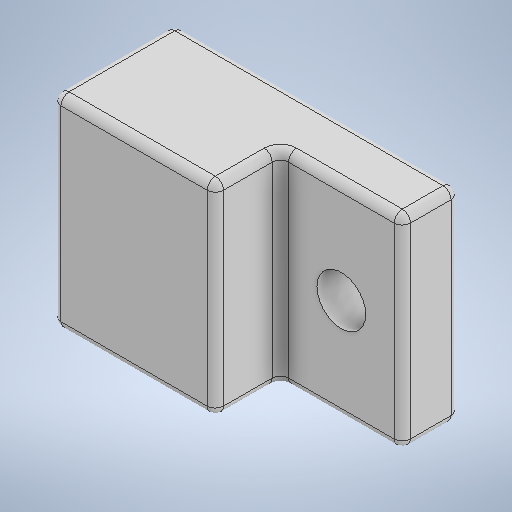
# Autodesk Inventor part: Holder
Saved by Autodesk Inventor 2025.1 (Build 291241000, 241)
## iProperties
Created: 2024-11-13
Part Number: Holder
Material: Genérico
Document SubType Name: Modeling
Designer: feror
Density: 1 g/cm^3
Appearance: Valor por defecto
Author: feror
Autodesk Inventor part; units mm, degrees
ref_plane "YZ Plane" through (0, 0, 0) normal (1, 0, 0) x (0, 1, 0)
ref_plane "XZ Plane" through (0, 0, 0) normal (0, 1, 0) x (-1, 0, 0)
ref_plane "XY Plane" through (0, 0, 0) normal (0, 0, 1) x (1, 0, 0)
sketch "Boceto1" plane through (0, 0, 0) normal (0, 0, 1) x (1, 0, 0)
  line L0 (0, 0) -> (35, 0)
  line L1 (35, 0) -> (35, 25)
  line L2 (35, 25) -> (0, 25)
  line L3 (0, 25) -> (0, 0)
  dimension "d0" = 35
  dimension "d1" = 25
  constraints: 8 end point, 2 parallel, 1 horizontal, 1 perpendicular
  measures "d0" distance of L2.end L1.end
  measures "d1" distance of L1.end L0.end
extrude "Extrusión1" add sketch "Boceto1" along normal blind 15
sketch "Boceto2" plane through (0, 0, 15) normal (0, 0, 1) x (1, 0, 0)
  line L0 (35, 0) -> (35, 25) projected
  line L1 (35, 25) -> (0, 25) projected
  line L2 (35, 0) -> (20, 0)
  line L3 (20, 0) -> (20, 25)
  line L4 (20, 25) -> (35, 25)
  line L5 (35, 25) -> (35, 0)
  point P0 (0, 0)
  dimension "d4" = 15
  constraints: 8 end point, 2 parallel, 1 horizontal, 1 perpendicular, 1 point on line
  measures "d4" distance of L3.end L4.end
extrude "Extrusión2" cut sketch "Boceto2" against normal blind 8
fillet "Empalme1" radius 1 18 edges at (20, 25, 11) (20, 12.5, 15) (27.5, 25, 7) (20, 12.5, 7) (35, 12.5, 7) (35, 25, 3.5) (35, 12.5, 0) (17.5, 25, 0) (10, 25, 15) (0, 25, 7.5) (0, 12.5, 15) (10, 0, 15) (20, 0, 11) (27.5, 0, 7) (35, 0, 3.5) (17.5, 0, 0) (0, 0, 7.5) (0, 12.5, 0)
sketch "Boceto3" plane through (0, 0, 7) normal (0, 0, 1) x (1, 0, 0)
  point P0 (0, 0)
sketch "Boceto4" plane through (0, 0, 7) normal (0, 0, 1) x (1, 0, 0)
  line L0 (21, 24) -> (34, 24) projected
  line L1 (27.5, 24) -> (27.5, 12.5)
  line L2 (27.5, 12.5) -> (34, 12.5)
  circle A0 centre (27.5, 12.5) radius 3
  point P0 (0, 0)
  dimension "d8" = 11.5
  dimension "d9" = 6
  constraints: 4 end point, 1 centre point, 1 coincident, 1 midpoint, 1 perpendicular, 1 vertical
  measures "d8" distance of L1.start L1.end
  measures "d9" diameter of A0
sketch "Boceto5" plane through (0, 0, 7) normal (0, 0, 1) x (1, 0, 0)
  point P0 (0, 0)
extrude "Extrusión3" cut sketch "Boceto4" against normal blind 8
sketch "Boceto6" plane through (0, 1, 1) normal (-1, 0, 0) x (0, 0, 1)
  line L0 (13, 0) -> (13, 23) projected
  line L1 (13, 11.5) -> (6.5, 11.5)
  circle A0 centre (6.5, 11.5) radius 3
  point P0 (-1, -1)
  dimension "d12" = 6.5
  dimension "d13" = 6
  constraints: 2 end point, 1 centre point, 1 coincident, 1 horizontal, 1 midpoint
  measures "d12" distance of L1.start L1.end
  measures "d13" diameter of A0
extrude "Extrusión4" cut sketch "Boceto6" against normal blind 10
sketch "Boceto7" plane through (0, 1, 1) normal (-1, 0, 0) x (0, 0, 1)
  point P0 (-1, -1)
